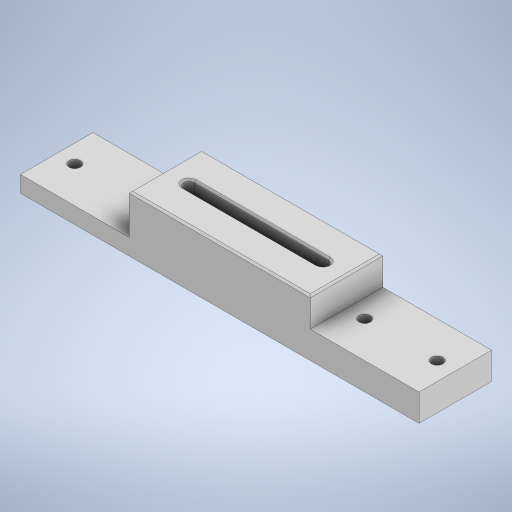
# Autodesk Inventor part: middle_hole
Saved by Autodesk Inventor 2023 (Build 270158000, 158)
## iProperties
Created: 2023-11-20
Part Number: middle_hole
Material: Všeobecné
Document SubType Name: Modeling
Designer: zavrel
Density: 1 g/cm^3
Appearance: Výchozí
Author: zavrel
Autodesk Inventor part; units mm, degrees
ref_plane "YZ Plane" through (0, 0, 0) normal (1, 0, 0) x (0, 1, 0)
ref_plane "XZ Plane" through (0, 0, 0) normal (0, 1, 0) x (-1, 0, 0)
ref_plane "XY Plane" through (0, 0, 0) normal (0, 0, 1) x (1, 0, 0)
sketch "Náčrt1" plane through (0, 0, 0) normal (0, 1, 0) x (-1, 0, 0)
  line L0 (0, 0) -> (110, 0)
  line L1 (110, 0) -> (110, -20)
  line L2 (110, -20) -> (0, -20)
  line L3 (0, -20) -> (0, 0)
  line L4 (55, -20) -> (55, 0) construction
  line L5 (36.5, -10) -> (73.5, -10) construction
  line L6 (36.5, -11.5) -> (73.5, -11.5)
  line L7 (73.5, -8.5) -> (36.5, -8.5)
  arc A0 (36.5, -8.5) -> (36.5, -11.5) centre (36.5, -10) ccw
  arc A1 (73.5, -11.5) -> (73.5, -8.5) centre (73.5, -10) ccw
  line L8 (110, -10) -> (0, -10) construction
  circle A2 centre (105, -10) radius 1.6
  circle A3 centre (85, -10) radius 1.6
  circle A4 centre (5, -10) radius 1.6
  circle A5 centre (25, -10) radius 1.6
  point P0 (55, -10)
  point P1 (35, -10)
  point P2 (75, -10)
  dimension "d0" = 20
  dimension "d1" = 110
  dimension "d2" = 3
  dimension "d3" = 40
  dimension "d4" = 3.2
  dimension "d6" = 25
  dimension "d7" = 5
  constraints: 20 end point, 6 centre point, 6 midpoint, 6 point on circle, 4 tangent, 3 parallel, 2 perpendicular, 2 point on line, 2 symmetric about line, 1 equal radius, 1 horizontal, 2 other
  measures "d0" distance between parallel lines of L2 L0
  measures "d1" distance of L1.end L2.end
  measures "d2" distance between parallel lines of L6 L7
  measures "d3" distance of point (35, -10) point (75, -10)
  measures "d4" diameter of A2
  measures "d6" distance from line of L1 A3.centre
  measures "d7" distance from line of L1 A2.centre
extrude "Vysunutí1" add sketch "Náčrt1" along normal blind 16
sketch "Náčrt2" plane through (0, 16, 0) normal (0, 1, 0) x (1, 0, 0)
  line L0 (0, 20) -> (-110, 20) projected
  line L1 (-110, 20) -> (-110, 0) projected
  line L2 (-110, 0) -> (0, 0) projected
  line L3 (0, 0) -> (0, 20) projected
  arc A0 (-36.5, 8.5) -> (-36.5, 11.5) centre (-36.5, 10) ccw projected
  line L4 (-36.5, 8.5) -> (-73.5, 8.5) projected
  arc A1 (-73.5, 11.5) -> (-73.5, 8.5) centre (-73.5, 10) ccw projected
  line L5 (-73.5, 11.5) -> (-36.5, 11.5) projected
  circle A2 centre (-25, 10) radius 1.6 projected
  circle A3 centre (-5, 10) radius 1.6 projected
  circle A4 centre (-85, 10) radius 1.6 projected
  circle A5 centre (-105, 10) radius 1.6 projected
  line L6 (-80, 0) -> (-80, 20)
  line L7 (-30, 0) -> (-30, 20)
  point P0 (0, 10)
  point P1 (-30, 10)
  dimension "d10" = 30
  dimension "d11" = 30
  constraints: 4 end point, 4 point on line, 2 midpoint, 2 parallel
  measures "d10" distance between parallel lines of L1 L6
  measures "d11" distance of point (0, 10) point (-30, 10)
extrude "Vysunutí2" cut sketch "Náčrt2" against normal blind 11 contours L6 L2 L1 L0
sketch "Náčrt3" plane through (0, 16, 0) normal (0, 1, 0) x (1, 0, 0)
  circle A0 centre (-5, 10) radius 1.6 projected
  circle A1 centre (-25, 10) radius 1.6 projected
  arc A2 (-36.5, 8.5) -> (-36.5, 11.5) centre (-36.5, 10) ccw projected
  line L0 (-36.5, 8.5) -> (-73.5, 8.5) projected
  arc A3 (-73.5, 11.5) -> (-73.5, 8.5) centre (-73.5, 10) ccw projected
  line L1 (-73.5, 11.5) -> (-36.5, 11.5) projected
  line L2 (-80, 20) -> (-80, 0) projected
  line L3 (-80, 0) -> (0, 0) projected
  line L4 (0, 0) -> (0, 20) projected
  line L5 (0, 20) -> (-80, 20) projected
  line L6 (-30, 0) -> (-30, 20)
  dimension "d14" = 30
  constraints: 2 end point, 2 point on line, 1 perpendicular
  measures "d14" distance between parallel lines of L4 L6
extrude "Vysunutí3" cut sketch "Náčrt3" against normal blind 8 contours L5 L4 L3 L6
sketch "Náčrt4" plane through (0, 0, 0) normal (0, -1, 0) x (1, 0, 0)
  line L0 (0, -20) -> (-110, -20) projected
  line L1 (0, 0) -> (0, -20) projected
  line L2 (-110, 0) -> (0, 0) projected
  line L3 (-110, -20) -> (-110, 0) projected
  arc A0 (-36.5, -11.5) -> (-36.5, -8.5) centre (-36.5, -10) ccw projected
  line L4 (-73.5, -11.5) -> (-36.5, -11.5) projected
  arc A1 (-73.5, -8.5) -> (-73.5, -11.5) centre (-73.5, -10) ccw projected
  line L5 (-36.5, -8.5) -> (-73.5, -8.5) projected
  circle A2 centre (-25, -10) radius 1.6 projected
  circle A3 centre (-5, -10) radius 1.6 projected
  circle A4 centre (-85, -10) radius 1.6 projected
  circle A5 centre (-105, -10) radius 1.6 projected
  circle A6 centre (-105, -10) radius 1.6 projected
  line L6 (-105, -6.8246) -> (-102.25, -8.4123)
  line L7 (-102.25, -8.4123) -> (-102.25, -11.5877)
  line L8 (-102.25, -11.5877) -> (-105, -13.1754)
  line L9 (-105, -13.1754) -> (-107.75, -11.5877)
  line L10 (-107.75, -11.5877) -> (-107.75, -8.4123)
  line L11 (-107.75, -8.4123) -> (-105, -6.8246)
  circle A7 centre (-85, -10) radius 1.6 projected
  line L12 (-84.9134, -6.8258) -> (-82.2077, -8.4879)
  line L13 (-82.2077, -8.4879) -> (-82.2943, -11.6621)
  line L14 (-82.2943, -11.6621) -> (-85.0866, -13.1742)
  line L15 (-85.0866, -13.1742) -> (-87.7923, -11.5121)
  line L16 (-87.7923, -11.5121) -> (-87.7057, -8.3379)
  line L17 (-87.7057, -8.3379) -> (-84.9134, -6.8258)
  circle A8 centre (-25, -10) radius 1.6 projected
  line L18 (-24.9679, -6.8247) -> (-22.2341, -8.4401)
  line L19 (-22.2341, -8.4401) -> (-22.2662, -11.6154)
  line L20 (-22.2662, -11.6154) -> (-25.0321, -13.1753)
  line L21 (-25.0321, -13.1753) -> (-27.7659, -11.5599)
  line L22 (-27.7659, -11.5599) -> (-27.7338, -8.3846)
  line L23 (-27.7338, -8.3846) -> (-24.9679, -6.8247)
  circle A9 centre (-5, -10) radius 1.6 projected
  line L24 (-4.9763, -6.8247) -> (-2.2382, -8.4328)
  line L25 (-2.2382, -8.4328) -> (-2.2619, -11.6082)
  line L26 (-2.2619, -11.6082) -> (-5.0237, -13.1753)
  line L27 (-5.0237, -13.1753) -> (-7.7618, -11.5672)
  line L28 (-7.7618, -11.5672) -> (-7.7381, -8.3918)
  line L29 (-7.7381, -8.3918) -> (-4.9763, -6.8247)
  point P0 (-102.25, -10)
  point P1 (-107.75, -10)
  dimension "d17" = 5.5
  constraints: 48 end point, 4 coincident, 3 equal length, 2 midpoint, 52 other
  measures "d17" distance of point (-102.25, -10) point (-107.75, -10)
extrude "Vysunutí4" cut sketch "Náčrt4" against normal blind 2.5 contours L6 L7 L8 L9 L10 L11 | L12 L13 L14 L15 L16 L17 | L18 L19 L20 L21 L22 L23 | L24 L25 L26 L27 L28 L29
chamfer "Zkosení1" distance 0.5 angle 45 16 edges at (-55, 16, -8.5) (-75, 16, -10) (-55, 16, -11.5) (-35, 16, -10) (-55, 16, 0) (-80, 16, -10) (-55, 16, -20) (-30, 16, -10) (-55, 0, 0) (-110, 0, -10) (-55, 0, -20) (0, 0, -10) (-55, 0, -11.5) (-35, 0, -10) (-55, 0, -8.5) (-75, 0, -10)
